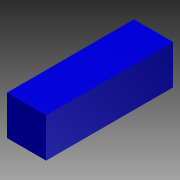
# Autodesk Inventor part: Turnigy2200mAh4S40C
Saved by Autodesk Inventor 2012 (Build 160160000, 160)
## iProperties
Created: 2012-03-28
Part Number: Turnigy2200mAh4S40C
Material: ABS Plastic
Document SubType Name: Modeling
Designer: Admin
Density: 2.03325 g/cm^3
Mass: 258.548 g
Surface Area: 172.72 cm^2
Volume: 127.16 cm^3
Author: Admin
Autodesk Inventor part; units mm, degrees
ref_plane "YZ Plane" through (0, 0, 0) normal (1, 0, 0) x (0, 1, 0)
ref_plane "XZ Plane" through (0, 0, 0) normal (0, 1, 0) x (-1, 0, 0)
ref_plane "XY Plane" through (0, 0, 0) normal (0, 0, 1) x (1, 0, 0)
sketch "Sketch1" plane through (0, 0, 0) normal (0, 0, 1) x (1, 0, 0)
  line L0 (0, 0) -> (-34, 0)
  line L1 (-34, 0) -> (-34, 34)
  line L2 (-34, 34) -> (0, 34)
  line L3 (0, 34) -> (0, 0)
  dimension "d0" = 34
  dimension "d1" = 34
  constraints: 8 end point, 2 parallel, 1 horizontal, 1 perpendicular
  measures "d0" distance of L1.end L2.end
  measures "d1" distance of L0.end L1.end
extrude "Extrusion1" add sketch "Sketch1" along normal blind 110
body "Solid1"
